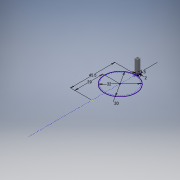
# Autodesk Inventor part: Part3
Saved by Autodesk Inventor 2016 (Build 200138000, 138)
## iProperties
Created: 2016-09-30
Part Number: Part3
Material: 一般
Document SubType Name: Modeling
Designer: KOTA-NPC2
Density: 1 g/cm^3
Appearance: 既定
Author: KOTA-NPC2
Autodesk Inventor part; units mm, degrees
ref_plane "YZ Plane" through (0, 0, 0) normal (1, 0, 0) x (0, 1, 0)
ref_plane "XZ Plane" through (0, 0, 0) normal (0, 1, 0) x (-1, 0, 0)
ref_plane "XY Plane" through (0, 0, 0) normal (0, 0, 1) x (1, 0, 0)
sketch "スケッチ1" plane through (0, 0, 0) normal (0, 0, 1) x (1, 0, 0)
  circle A0 centre (0, 30) radius 16
  circle A1 centre (0, 48) radius 1
  line L0 (0, 67.2165) -> (0, -64.9114) construction
  circle A2 centre (0, 30) radius 15 construction
  line L1 (1.5, 49.5) -> (-1.5, 49.5)
  line L2 (-1.5, 49.5) -> (-1.5, 46.5)
  line L3 (-1.5, 46.5) -> (1.5, 46.5)
  line L4 (1.5, 46.5) -> (1.5, 49.5)
  line L5 (1.5, 46.5) -> (1.5, 45.9295)
  line L6 (-1.5, 46.5) -> (-1.5, 45.9295)
  circle A3 centre (24, 11.1876) radius 1.05
  circle A4 centre (-24, 11.1876) radius 1.05
  line L7 (0, 30) -> (24, 11.1876) construction
  line L8 (0, 30) -> (-24, 11.1876) construction
  point P0 (0, 0)
  dimension "d0" = 32
  dimension "d1" = 2
  dimension "d2" = 1
  dimension "d3" = 30
  dimension "d4" = 30
  dimension "d5" = 3
  dimension "d6" = 3
  dimension "d7" = 46.5
  dimension "d8" = 1.5
  constraints: 18 end point, 5 centre point, 3 parallel, 3 point on line, 2 point on circle, 2 vertical, 1 coincident, 1 horizontal, 1 perpendicular, 4 other
  measures "d0" diameter of A0
  measures "d1" diameter of A1
  measures "d3" distance of point (0, 0) A0.centre
  measures "d4" diameter of A2
  measures "d5" distance of L1.start L1.end
  measures "d6" distance of L3.end L1.start
  measures "d7" distance from line of point (0, 0) L3
  measures "d8" distance between parallel lines of L0 L4
extrude "押し出し1" add sketch "スケッチ1" against normal blind 14 contours L3 L2 L1 L4 | A1
extrude "押し出し3" cut sketch "スケッチ1" against normal blind 2 contours A1
